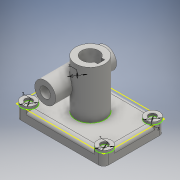
# Autodesk Inventor part: 240626_part3
Saved by Autodesk Inventor 2016 (Build 200138000, 138)
## iProperties
Created: 2024-06-26
Part Number: 240626_part3
Material: 일반
Document SubType Name: Modeling
Designer: pc
Density: 1 g/cm^3
Appearance: 기본값
Author: pc
Autodesk Inventor part; units mm, degrees
ref_plane "YZ Plane" through (0, 0, 0) normal (1, 0, 0) x (0, 1, 0)
ref_plane "XZ Plane" through (0, 0, 0) normal (0, 1, 0) x (-1, 0, 0)
ref_plane "XY Plane" through (0, 0, 0) normal (0, 0, 1) x (1, 0, 0)
sketch "스케치1" plane through (0, 0, 0) normal (0, 0, 1) x (1, 0, 0)
  line L0 (18.1179, -12.6078) -> (-18.1179, -12.6078)
  line L1 (-18.1179, -12.6078) -> (-18.1179, 12.6078)
  line L2 (-18.1179, 12.6078) -> (18.1179, 12.6078)
  line L3 (18.1179, 12.6078) -> (18.1179, -12.6078)
  line L4 (18.1179, -12.6078) -> (-18.1179, 12.6078) construction
  line L5 (-18.1179, -12.6078) -> (18.1179, 12.6078) construction
  point P0 (0, 0)
  constraints: 12 end point, 2 midpoint, 2 parallel, 1 horizontal, 1 perpendicular
extrude "돌출1" add sketch "스케치1" along normal blind 5
sketch "스케치2" plane through (0, 0, 5) normal (0, 0, 1) x (1, 0, 0)
  circle A0 centre (-15.5331, 10.141) radius 3
  circle A1 centre (-15.5331, -10.025) radius 3
  circle A2 centre (15.8794, -10.025) radius 3
  circle A3 centre (15.6354, 10.141) radius 3
  line L0 (-18.1179, 12.6078) -> (-18.1179, -12.6078) projected
  line L1 (18.1179, 12.6078) -> (-18.1179, 12.6078) projected
  line L2 (-18.1179, -12.6078) -> (18.1179, -12.6078) projected
  line L3 (18.1179, -12.6078) -> (18.1179, 12.6078) projected
  circle A4 centre (0, 0) radius 6.0442
  arc A5 (3.234, 1.4702) -> (3.234, -1.4702) centre (0, 0) ccw
  line L4 (4.5625, 1.4702) -> (3.234, 1.4702)
  line L5 (3.234, -1.4702) -> (4.5625, -1.4702)
  line L6 (4.5625, -1.4702) -> (4.5625, 1.4702)
  line L7 (4.5625, 1.4702) -> (2.5426, -1.4702) construction
  line L8 (2.5426, 1.4702) -> (4.5625, -1.4702) construction
  circle A6 centre (15.6354, 10.141) radius 1.5
  circle A7 centre (-15.5331, 10.141) radius 1.5
  circle A8 centre (-15.5331, -10.025) radius 1.5
  circle A9 centre (15.8794, -10.025) radius 1.5
  dimension "d2" = 6
  dimension "d3" = 6
  dimension "d4" = 6
  dimension "d5" = 6
  dimension "d6" = 3
  dimension "d7" = 3
  dimension "d8" = 3
  dimension "d9" = 3
  constraints: 10 centre point, 10 end point, 6 coincident, 2 point on circle, 1 horizontal, 1 parallel
  measures "d2" diameter of A0
  measures "d3" diameter of A1
  measures "d4" diameter of A2
  measures "d5" diameter of A3
  measures "d6" diameter of A6
  measures "d7" diameter of A7
  measures "d8" diameter of A8
  measures "d9" diameter of A9
extrude "돌출2" add sketch "스케치2" along normal blind 1 contours A0 L0 L1 | L1 A0 | A0 L0 | L1 A3 L3 | A3 L1 | L0 A1 | A1 L2 L0 | L3 A3 | L3 A2 L2 | A2 L3 | A1 L2 | L2 A2 picked at (-15.5934, 12.2819) picked at (15.5751, 12.2819) picked at (-15.4728, -12.2432) picked at (15.8191, -12.2432)
extrude "돌출3" add sketch "스케치2" along normal blind 20 contours A4
fillet "모깎기1" radius 2 4 edges at (-18.1179, -12.6078, 2.5) (-18.1179, 12.6078, 2.5) (18.1179, 12.6078, 2.5) (18.1179, -12.6078, 2.5)
sketch "스케치3" plane through (0, 0, 5) normal (0, 0, 1) x (1, 0, 0)
  point P0 (0, 0)
fillet "모깎기2" radius 2 4 edges at (0.0511, 12.6078, 5) (-18.1179, 0.058, 5) (18.1179, 0.2144, 5) (0.1731, -12.6078, 5)
sketch "스케치4" plane through (-16.1179, 12.6078, 0) normal (0, 1, 0) x (1, 0, 0)
  line L0 (10.0737, -5) -> (10.0737, -25) projected
  circle A0 centre (10.0737, -15) radius 4.3611
  circle A1 centre (10.0737, -15) radius 2.194
  point P0 (16.1179, 0)
  constraints: 2 centre point, 1 coincident, 1 midpoint
extrude "돌출4" add sketch "스케치4" against normal up to surface (25.2156 mm away) contours A0 L0 A1 | L0 A1 A0
